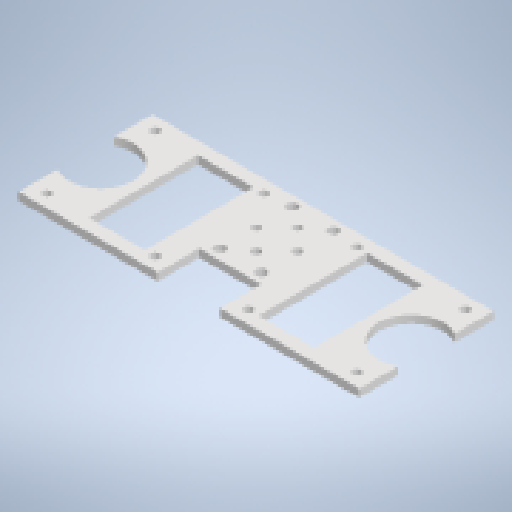
# Autodesk Inventor part: hipjoint_upper
Saved by Autodesk Inventor 2024.1 (Build 281209000, 209)
## iProperties
Created: 2024-10-09
Part Number: hipjoint_upper
Material: 一般
Document SubType Name: Sheet Metal
Designer: hibik
Density: 1 g/cm^3
Sheet Metal Rule: Default_mm
Appearance: 既定
Author: hibik
Autodesk Inventor part; units mm, degrees
ref_plane "YZ Plane" through (0, 0, 0) normal (1, 0, 0) x (0, 1, 0)
ref_plane "XZ Plane" through (0, 0, 0) normal (0, 1, 0) x (-1, 0, 0)
ref_plane "XY Plane" through (0, 0, 0) normal (0, 0, 1) x (1, 0, 0)
sketch "スケッチ1" plane through (0, 0, 0) normal (0, 1, 0) x (-1, 0, 0)
  circle A0 centre (30, 0) radius 6.25
  circle A1 centre (-30, 0) radius 6.25
  line L0 (30, -13) -> (6, -13)
  line L1 (6, -13) -> (6, 13)
  line L2 (6, 13) -> (30, 13)
  line L3 (30, 13) -> (30, -13)
  line L4 (-30, -13) -> (-6, -13)
  line L5 (-6, -13) -> (-6, 13)
  line L6 (-6, 13) -> (-30, 13)
  line L7 (-30, 13) -> (-30, -13) construction
  line L8 (0, -18.2) -> (0, 18.2)
  line L9 (30, -13) -> (33, -13)
  line L10 (33, -13) -> (33, 13)
  line L11 (33, 13) -> (30, 13)
  line L12 (30, 13) -> (30, -13) construction
  line L13 (-30, -13) -> (-33, -13)
  line L14 (-33, -13) -> (-33, 13)
  line L15 (-33, 13) -> (-30, 13)
  line L16 (-30, 13) -> (-30, -13)
  line L17 (6, -13) -> (-6, -13)
  line L18 (-6, -13) -> (-6, 13)
  line L19 (-6, 13) -> (6, 13)
  line L20 (6, 13) -> (6, -13)
  line L21 (50.75, 0) -> (-50.75, 0)
  point P0 (0, 0)
  point P1 (33, -5.4829)
  point P2 (33, 5.4829)
  point P3 (-33, 5.4829)
  point P4 (-33, -5.4829)
  dimension "d0" = 12.5
  dimension "d1" = 12.5
  dimension "d2" = 24
  dimension "d3" = 26
  dimension "d4" = 24
  dimension "d5" = 26
  dimension "d6" = 60
  dimension "d7" = 3
  dimension "d8" = 3
  measures "d0" diameter of A0
  measures "d1" diameter of A1
  measures "d2" distance of L1.end L2.end
  measures "d3" distance of L0.end L1.end
  measures "d4" distance of L6.end L5.end
  measures "d5" distance of L5.end L4.end
  measures "d6" distance of A1.centre A0.centre
  measures "d7" distance of L11.end L10.end
  measures "d8" distance of L14.end L15.end
extrude "プレート1" add sketch "スケッチ1" along normal blind 1.5 contours A0 L3 L11 L10 | L10 L9 L3 A0 | A0 L21 L1 L2 L3 | L3 L0 L1 L21 A0 | L21 L8 L19 L1 | L1 L17 L8 L21 | L21 L5 L19 L8 | L8 L17 L5 L21 | L21 A1 L16 L6 L5 | L5 L4 L16 A1 L21 | L16 A1 L14 L15 | L13 L14 A1 L16
sketch "スケッチ2" plane through (0, 1.5, 0) normal (0, 1, 0) x (1, 0, 0)
  circle A0 centre (-30, 10.5) radius 0.85 projected
  circle A1 centre (-9, 10.5) radius 0.85 projected
  circle A2 centre (-9, -10.5) radius 0.85 projected
  circle A3 centre (-30, -10.5) radius 0.85 projected
  circle A4 centre (9, -10.5) radius 0.85 projected
  circle A5 centre (30, -10.5) radius 0.85 projected
  circle A6 centre (30, 10.5) radius 0.85 projected
  circle A7 centre (9, 10.5) radius 0.85 projected
  line L0 (30, -10.5) -> (9, -10.5)
  line L1 (9, -10.5) -> (9, 10.5) construction
  line L2 (9, 10.5) -> (30, 10.5)
  line L3 (30, 10.5) -> (30, -10.5) construction
  line L4 (-9, -10.5) -> (-30, -10.5)
  line L5 (-30, -10.5) -> (-30, 10.5) construction
  line L6 (-30, 10.5) -> (-9, 10.5)
  line L7 (-9, 10.5) -> (-9, -10.5) construction
  line L8 (21.75, -10.5) -> (11, -10.5)
  line L9 (11, -10.5) -> (11, 10.5)
  line L10 (11, 10.5) -> (21.75, 10.5)
  line L11 (21.75, 10.5) -> (21.75, -10.5)
  line L12 (-11, -10.5) -> (-21.75, -10.5)
  line L13 (-21.75, -10.5) -> (-21.75, 10.5)
  line L14 (-21.75, 10.5) -> (-11, 10.5)
  line L15 (-11, 10.5) -> (-11, -10.5)
  arc A8 (33, 5.4829) -> (33, -5.4829) centre (30, 0) ccw projected
  arc A9 (-33, -5.4829) -> (-33, 5.4829) centre (-30, 0) ccw projected
  line L16 (33, -13) -> (-33, -13) projected
  line L17 (33, -5.4829) -> (33, -13) projected
  arc A10 (33, 5.4829) -> (33, -5.4829) centre (30, 0) ccw projected
  line L18 (33, 13) -> (33, 5.4829) projected
  line L19 (-33, 13) -> (33, 13) projected
  line L20 (-33, 5.4829) -> (-33, 13) projected
  arc A11 (-33, -5.4829) -> (-33, 5.4829) centre (-30, 0) ccw projected
  line L21 (-33, -13) -> (-33, -5.4829) projected
  line L22 (-6, -13) -> (6, -13)
  line L23 (6, -13) -> (6, -5)
  line L24 (6, -5) -> (-6, -5)
  line L25 (-6, -5) -> (-6, -13)
  line L26 (0, 18.2) -> (0, -18.2) projected
  point P0 (0, 0)
  dimension "d15" = 2
  dimension "d16" = 2
  dimension "d17" = 8.25
  dimension "d18" = 8.25
  dimension "d21" = 8
  dimension "d22" = 12
  constraints: 40 end point, 10 parallel, 5 horizontal, 5 perpendicular, 5 point on line, 1 other
  measures "d15" distance between parallel lines of L1 L9
  measures "d16" distance between parallel lines of L7 L15
  measures "d17" distance from line of L11 A8.centre
  measures "d18" distance from line of A9.centre L13
  measures "d21" distance of L24.end L22.start
  measures "d22" distance of L23.end L24.end
extrude "切り取り1" cut sketch "スケッチ2" against normal blind 1.5 contours A0 | A1 | A2 | A3 | A4 | A5 | A6 | A7 | L0 L9 L2 L11 | L4 L13 L6 L15 | L16 L26 L24 L23 | L26 L16 L25 L24
sketch "スケッチ3" plane through (0, 1.5, 0) normal (0, 1, 0) x (1, 0, 0)
  line L0 (-6, -5) -> (-6, -13) projected
  line L1 (-33, 13) -> (33, 13) projected
  line L2 (-6, -5) -> (6, -5) construction
  line L3 (6, -5) -> (6, 13) construction
  line L4 (6, 13) -> (-6, 13)
  line L5 (-6, 13) -> (-6, -5) construction
  line L6 (6, -5) -> (6, -13) projected
  circle A0 centre (-4, 11) radius 1
  circle A1 centre (4, 11) radius 1
  circle A2 centre (4, -3) radius 1
  circle A3 centre (-4, -3) radius 1
  line L7 (0, 19.4) -> (0, -18.4) projected
  circle A4 centre (0, 4) radius 7.0623 construction
  circle A5 centre (0, 4) radius 4 construction
  circle A6 centre (0, 8) radius 0.8
  circle A7 centre (-4, 4) radius 0.8
  circle A8 centre (0, 0) radius 0.8
  circle A9 centre (4, 4) radius 0.8
  point P0 (0, 0)
  dimension "d27" = 8
  dimension "d23" = 2
  dimension "d24" = 8
  dimension "d25" = 14
  dimension "d26" = 2
  dimension "d28" = 1.6
  dimension "d31" = 360
  constraints: 9 centre point, 8 end point, 3 equal radius, 3 point on line, 3 vertical alignment, 2 horizontal alignment, 2 parallel, 2 tangent, 1 coincident, 1 collinear, 1 horizontal, 1 perpendicular, 1 symmetric about line, 11 other
  measures "d23" diameter of A0
  measures "d24" distance of A1.centre A0.centre
  measures "d25" distance of A1.centre A2.centre
  measures "d26" distance from line of L1 A1.centre
  measures "d28" diameter of A6
extrude "切り取り2" cut sketch "スケッチ3" against normal blind 1.5
equation "\"d16\" = d15"
equation "\"d18\" = d17"
equation "\"d19\" = Thickness"
equation "\"d33\" = Thickness"
equation "\"d9\" = Thickness"
equation "\"BendRadius\" = Thickness"
equation "\"BendReliefWidth\" = Thickness"
equation "\"BendReliefDepth\" = 0.5 * Thickness"
equation "\"CornerReliefSize\" = 4 * Thickness"
equation "\"MinimumRemnant\" = 2 * Thickness"
equation "\"TransitionRadius\" = BendRadius"
equation "\"JacobiRadiusSize\" = BendRadius"
equation "\"GapSize\" = Thickness"
equation "\"Thickness\" = 1.5"
